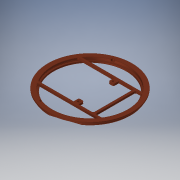
# Autodesk Inventor part: ODroid Holder-40x
Saved by Autodesk Inventor 2018 (Build 220112000, 112)
## iProperties
Part Number: ODroid Holder-40x
Material: Kupfer
Document SubType Name: Modeling
Designer: Jochen Alt
Mass: 179.761 g
Surface Area: 193.281 cm^2
Volume: 20.1075 cm^3
Density: 8.94 g/cm^3
Appearance: Kupfer - satiniert
Author: Jochen Alt
Autodesk Inventor part; units mm, degrees
ref_plane "YZ Plane" through (0, 0, 0) normal (1, 0, 0) x (0, 1, 0)
ref_plane "XZ Plane" through (0, 0, 0) normal (0, 1, 0) x (-1, 0, 0)
ref_plane "XY Plane" through (0, 0, 0) normal (0, 0, 1) x (1, 0, 0)
sketch "Skizze1" plane through (0, 0, 0) normal (0, 0, 1) x (1, 0, 0)
  circle A0 centre (0, 0) radius 59
  circle A1 centre (0, 0) radius 53
  circle A2 centre (0, 0) radius 54 construction
  line L0 (-82.81, 0) -> (83.86, 0) construction
  line L1 (34.0421, -45.718) -> (-0.6682, -56.9961)
  line L2 (-54.413, 16.9772) -> (-32.9608, 46.5036)
  line L3 (-0.6682, 56.9961) -> (34.0421, 45.718)
  line L4 (-32.9608, -46.5036) -> (-54.413, -16.9772)
  arc A3 (-32.9608, -46.5036) -> (-0.6682, -56.9961) centre (0, 0) ccw
  arc A4 (-54.413, 16.9772) -> (-54.413, -16.9772) centre (0, 0) ccw
  arc A5 (34.0421, -45.718) -> (34.0421, 45.718) centre (0, 0) ccw
  arc A6 (-0.6682, 56.9961) -> (-32.9608, 46.5036) centre (0, 0) ccw
  circle A7 centre (0, 0) radius 46.9646
  point P0 (60.05, 0)
  dimension "d7" = 118
  dimension "d100" = 106
  dimension "d108" = 108
  dimension "d110" = 57
  dimension "d115" = 6.0354
  constraints: 8 centre point, 8 end point, 8 point on circle, 6 coincident, 3 concentric, 3 tangent, 2 other
  measures "d7" diameter of A0
  measures "d100" diameter of A1
  measures "d108" diameter of A2
  measures "d110" radius of A5
  measures "d115" radial gap between concentric circles of A7 A1
extrude "Extrusion3" add sketch "Skizze1" against normal blind 4 contours L1 A3 L4 A4 L2 A6 L3 A5
extrude "Extrusion4" add sketch "Skizze1" along normal blind 1.5 contours A0 | L1 A3 L4 A4 L2 A6 L3 A5
sketch "ODroidskizze" plane through (0, 0, 1.5) normal (0, 0, 1) x (1, 0, 0)
  line L0 (0, -82.6) -> (0, 82.6) construction
  line L1 (-82.6, 0) -> (82.6, 0) construction
  line L2 (8.7, -24.5009) -> (-49.3, -24.5009) construction
  line L3 (-49.3, -24.5009) -> (-49.3, 24.4991) construction
  line L4 (-49.3, 24.4991) -> (8.7, 24.4991) construction
  line L5 (8.7, 24.4991) -> (8.7, -24.5009) construction
  line L6 (8.7, -24.5009) -> (-49.3, 24.4991) construction
  line L7 (32.7, 28.2515) -> (32.7, -28.2515) construction
  line L8 (32.7, -28.2515) -> (-53.1741, 34.4377) construction
  line L9 (-53.1741, -34.4377) -> (32.7, 28.2515) construction
  line L10 (32.7, 26.2485) -> (32.7, -26.2515)
  line L11 (7.2, 20.7468) -> (10.2, 20.7468)
  line L12 (12.2, 22.7468) -> (12.2, 28.2515)
  line L13 (5.2, 28.2515) -> (5.2, 22.7468)
  line L14 (5.2, 20.7468) -> (12.2, 28.2515) construction
  line L15 (12.2, 20.7468) -> (5.2, 28.2515) construction
  line L16 (7.2, -20.7502) -> (10.2, -20.7502)
  line L17 (12.2, -22.7502) -> (12.2, -28.2515)
  line L18 (5.2, -28.2515) -> (5.2, -22.7502)
  line L19 (5.2, -20.7502) -> (12.2, -28.2515) construction
  line L20 (12.2, -20.7502) -> (5.2, -28.2515) construction
  arc A0 (5.2, 22.7468) -> (7.2, 20.7468) centre (7.2, 22.7468) ccw
  arc A1 (10.2, 20.7468) -> (12.2, 22.7468) centre (10.2, 22.7468) ccw
  arc A2 (12.2, -22.7502) -> (10.2, -20.7502) centre (10.2, -22.7502) ccw
  arc A3 (7.2, -20.7502) -> (5.2, -22.7502) centre (7.2, -22.7502) ccw
  arc A4 (32.7, 26.2485) -> (30.7, 28.2515) centre (30.7, 26.2515) ccw
  arc A5 (30.7, -28.2515) -> (32.7, -26.2515) centre (30.7, -26.2515) ccw
  line L21 (12.2, 28.2515) -> (30.7, 28.2515)
  line L22 (12.2, 28.2515) -> (32.7, 28.2515) construction
  line L23 (30.7, -28.2515) -> (12.2, -28.2515)
  line L24 (5.2, -28.2515) -> (-43.2559, -28.2515)
  line L25 (32.7, -28.2515) -> (12.2, -28.2515) construction
  line L26 (5.2, -28.2515) -> (-45.7943, -28.2515) construction
  circle A6 centre (0, 0) radius 59 projected
  circle A7 centre (0, 0) radius 53 projected
  circle A8 centre (0, 0) radius 53 projected
  arc A9 (-53.2754, -31.1581) -> (-53.2216, -31.25) centre (0, 0) ccw
  line L27 (-43.7135, 28.2515) -> (5.2, 28.2515)
  line L28 (-44.8425, 28.2515) -> (5.2, 28.2515) construction
  arc A10 (-45.4371, 27.266) -> (-44.9615, -27.2959) centre (0.2378, 0.3811) ccw
  arc A11 (-44.039, 31.25) -> (44.039, 31.25) centre (0, 0) ccw
  line L29 (-44.039, 31.25) -> (44.039, 31.25)
  line L30 (-44.039, -31.25) -> (44.039, -31.25)
  line L31 (35.7, -26.25) -> (35.7, 26.25)
  line L32 (37.7, 28.25) -> (43.7257, 28.25)
  arc A12 (45.4404, -27.2794) -> (45.4404, 27.2794) centre (0, 0) ccw
  line L33 (43.7257, -28.25) -> (37.7, -28.25)
  arc A13 (37.7, 28.25) -> (35.7, 26.25) centre (37.7, 26.25) ccw
  arc A14 (45.4404, 27.2794) -> (43.7257, 28.25) centre (43.7257, 26.25) ccw
  arc A15 (43.7257, -28.25) -> (45.4404, -27.2794) centre (43.7257, -26.25) ccw
  arc A16 (35.7, -26.25) -> (37.7, -28.25) centre (37.7, -26.25) ccw
  arc A17 (-43.7135, 28.2515) -> (-45.4371, 27.266) centre (-43.7135, 26.2515) ccw
  arc A18 (-44.9615, -27.2959) -> (-43.2559, -28.2515) centre (-43.2559, -26.2515) ccw
  point P0 (0.9483, -27.9891)
  point P1 (-20.301, 0)
  point P2 (-20.301, 0)
  point P3 (-6, 0)
  point P4 (44.0485, 0)
  point P5 (-44.3623, -28.2515)
  point P6 (44.8435, -28.25)
  point P7 (44.8435, 28.25)
  dimension "d30" = 49
  dimension "d31" = 58
  dimension "d38" = 6
  dimension "d39" = 7
  dimension "d40" = 7
  dimension "d62" = 108
  dimension "d69" = 3
  dimension "d70" = 2
  dimension "d72" = 2
  dimension "d114" = 5.2
  constraints: 64 end point, 40 point on circle, 25 tangent, 20 point on line, 16 centre point, 13 parallel, 10 horizontal, 9 equal radius, 7 coincident, 6 perpendicular, 5 midpoint, 1 other
  measures "d30" distance between parallel lines of L2 L4
  measures "d31" distance between parallel lines of L5 L3
  measures "d38" distance from line of L0 point (-6, 0)
  measures "d39" distance between parallel lines of L12 L13
  measures "d40" distance between parallel lines of L17 L18
  measures "d62" diameter of A11
  measures "d69" distance between parallel lines of L31 L10
  measures "d70" radius of A13
  measures "d72" radius of A17
  measures "d114" distance between parallel lines of L13 L0
extrude "Extrusion5" add sketch "ODroidskizze" against normal blind 2.5 contours A7 L29 A11 L30 | A14 L32 A13 L31 A16 L33 A15 A7 L30 L29 | A7 L30 A11 L29
hole "Bohrung1" at (8.7, 24.4991, 1.5) at (8.7, -24.5009, 1.5) direction (0, 0, -1) diameter 3.2 end through all
sketch "Skizze4" plane through (0, 0, -4) normal (0, 0, -1) x (-1, 0, 0)
  circle A0 centre (0, 0) radius 51
  circle A1 centre (0, 0) radius 53.0797
  dimension "d80" = 102
  constraints: 2 centre point, 2 coincident
  measures "d80" diameter of A0
extrude "Extrusion6" add sketch "Skizze4" against normal blind 2
ref_plane "Arbeitsebene1" through (0, 0, -1) normal (0, 0, 1) x (1, 0, 0)
sketch "Skizze8" plane through (0, 0, 1.5) normal (0, 0, 1) x (1, 0, 0)
  arc A0 (42.807, 31.25) -> (-42.807, 31.25) centre (0, 0) ccw construction
  arc A1 (-42.807, -31.25) -> (42.807, -31.25) centre (0, 0) ccw construction
  circle A2 centre (-18.1271, -49.8037) radius 2
  circle A3 centre (-18.1271, 49.8037) radius 2
  line L0 (-82.6, 0) -> (82.6, 0) construction
  point P0 (-53.0797, 0)
  dimension "d116" = 4
  dimension "d117" = 4
  constraints: 2 centre point, 2 point on circle, 1 point on line
  measures "d116" diameter of A2
  measures "d117" diameter of A3
extrude "Lidar-Holder-Nose" cut sketch "Skizze8" against normal blind 2.5
chamfer "Fase5" distance 0.5 angle 45 8 edges at (-43.6869, -31.7404, -4) (-57, 0, -4) (-17.614, -54.2102, -4) (-43.6869, 31.7404, -4) (-17.614, 54.2102, -4) (16.6869, 51.3571, -4) (57, 0, -4) (16.6869, -51.3571, -4)
